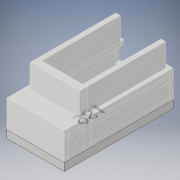
# Autodesk Inventor part: canBusHousing
Saved by Autodesk Inventor 2018.2 (Build 222227000, 227)
## iProperties
Created: 2017-12-01
Part Number: canBusHousing
Material: Generic
Document SubType Name: Modeling
Designer: steele
Density: 1 g/cm^3
Appearance: Default
Author: steele
Autodesk Inventor part; units mm, degrees
ref_plane "YZ Plane" through (0, 0, 0) normal (1, 0, 0) x (0, 1, 0)
ref_plane "XZ Plane" through (0, 0, 0) normal (0, 1, 0) x (-1, 0, 0)
ref_plane "XY Plane" through (0, 0, 0) normal (0, 0, 1) x (1, 0, 0)
sketch "Sketch1" plane through (6.5, -2.85, -13.25) normal (0, -1, 0) x (1, 0, 0)
  line L0 (-6.5, 13.25) -> (-6.5, -0.9821) construction
  line L1 (-6.5, 13.25) -> (1.0035, 13.25) construction
  line L2 (-14.0035, 27.4821) -> (-14.0035, -0.9821)
  line L3 (-14.0035, -0.9821) -> (1.0035, -0.9821)
  line L4 (1.0035, -0.9821) -> (1.0035, 27.4821)
  line L5 (1.0035, 27.4821) -> (-14.0035, 27.4821)
  line L6 (-14.0035, 27.4821) -> (1.0035, -0.9821) construction
  line L7 (-14.0035, -0.9821) -> (1.0035, 27.4821) construction
  constraints: 16 end point, 3 parallel, 2 midpoint, 1 horizontal, 1 perpendicular, 1 vertical
extrude "Extrusion1" add sketch "Sketch1" along normal blind 2
sketch "Sketch2" plane through (6.5, -4.85, -13.25) normal (0, -1, 0) x (1, 0, 0)
  line L0 (1.0035, 27.4821) -> (-14.0035, 27.4821) construction
  line L1 (-8.0035, 27.4821) -> (-8.0035, -0.9797) construction
  line L2 (-14.0035, 27.4821) -> (-14.0035, -0.9821) projected
  spline S0 degree 2 poles (-5.946, 16.5437) (-5.7113, 16.5437) (-5.3211, 16.3906) (-5.1803, 16.2572) knots 0 0 0 1 2 2 2
  spline S1 degree 2 poles (-5.1803, 16.2572) (-5.0444, 16.1312) (-4.8938, 15.7632) (-4.8938, 15.5755) knots 0 0 0 1 2 2 2
  spline S2 degree 2 poles (-4.8938, 15.5755) (-4.8938, 15.3655) (-5.0346, 15.0247) (-5.1679, 14.8987) knots 0 0 0 1 2 2 2
  spline S3 degree 2 poles (-5.1679, 14.8987) (-5.3359, 14.7406) (-5.8793, 14.5677) (-6.2967, 14.5677) knots 0 0 0 1 2 2 2
  spline S4 degree 2 poles (-6.2967, 14.5677) (-6.6747, 14.5677) (-7.3514, 14.7381) (-7.5762, 14.9036) knots 0 0 0 1 2 2 2
  spline S5 degree 2 poles (-7.5762, 14.9036) (-7.8133, 15.079) (-8.0628, 15.573) (-8.0628, 15.9336) knots 0 0 0 1 2 2 2
  spline S6 degree 2 poles (-8.0628, 15.9336) (-8.0628, 16.0151) (-8.0455, 16.2004) (-8.0208, 16.2794) knots 0 0 0 1 2 2 2
  line L3 (-8.0208, 16.2794) -> (-7.6281, 16.2794)
  line L4 (-7.6281, 16.2794) -> (-7.6281, 16.2597)
  spline S7 degree 2 poles (-7.6281, 16.2597) (-7.6577, 16.2078) (-7.7096, 15.9904) (-7.7096, 15.8793) knots 0 0 0 1 2 2 2
  spline S8 degree 2 poles (-7.7096, 15.8793) (-7.7096, 15.4791) (-7.181, 15.0222) (-6.6919, 14.9901) knots 0 0 0 1 2 2 2
  spline S9 degree 2 poles (-6.6919, 14.9901) (-6.8031, 15.1531) (-6.9044, 15.4495) (-6.9044, 15.6249) knots 0 0 0 1 2 2 2
  spline S10 degree 2 poles (-6.9044, 15.6249) (-6.9044, 15.7928) (-6.8303, 16.072) (-6.7241, 16.2127) knots 0 0 0 1 2 2 2
  spline S11 degree 2 poles (-6.7241, 16.2127) (-6.5981, 16.3758) (-6.2152, 16.5437) (-5.946, 16.5437) knots 0 0 0 1 2 2 2
  spline S12 degree 2 poles (-6.2053, 14.9802) (-5.8966, 14.9802) (-5.5063, 15.0938) (-5.4001, 15.1951) knots 0 0 0 1 2 2 2
  spline S13 degree 2 poles (-5.4001, 15.1951) (-5.3013, 15.284) (-5.2272, 15.4693) (-5.2272, 15.5779) knots 0 0 0 1 2 2 2
  spline S14 degree 2 poles (-5.2272, 15.5779) (-5.2272, 15.8299) (-5.5878, 16.1288) (-5.9287, 16.1288) knots 0 0 0 1 2 2 2
  spline S15 degree 2 poles (-5.9287, 16.1288) (-6.1214, 16.1288) (-6.3708, 16.03) (-6.4598, 15.9213) knots 0 0 0 1 2 2 2
  spline S16 degree 2 poles (-6.4598, 15.9213) (-6.524, 15.8422) (-6.566, 15.6471) (-6.566, 15.5335) knots 0 0 0 1 2 2 2
  spline S17 degree 2 poles (-6.566, 15.5335) (-6.566, 15.4026) (-6.4746, 15.1012) (-6.398, 14.9876) knots 0 0 0 1 2 2 2
  spline S18 degree 2 poles (-6.398, 14.9876) (-6.3684, 14.9851) (-6.2671, 14.9802) (-6.2053, 14.9802) knots 0 0 0 1 2 2 2
  spline S19 degree 2 poles (-8.0727, 13.2512) (-8.0727, 13.4784) (-7.9368, 13.8514) (-7.8109, 13.9823) knots 0 0 0 1 2 2 2
  spline S20 degree 2 poles (-7.8109, 13.9823) (-7.6874, 14.1108) (-7.3514, 14.2441) (-7.1612, 14.2441) knots 0 0 0 1 2 2 2
  spline S21 degree 2 poles (-7.1612, 14.2441) (-6.9142, 14.2441) (-6.4993, 13.9798) (-6.3758, 13.7279) knots 0 0 0 1 2 2 2
  line L5 (-6.3758, 13.7279) -> (-6.3634, 13.7279)
  spline S22 degree 2 poles (-6.3634, 13.7279) (-6.2325, 13.9527) (-5.9213, 14.17) (-5.6891, 14.17) knots 0 0 0 1 2 2 2
  spline S23 degree 2 poles (-5.6891, 14.17) (-5.3458, 14.17) (-4.8864, 13.6513) (-4.8864, 13.2512) knots 0 0 0 1 2 2 2
  spline S24 degree 2 poles (-4.8864, 13.2512) (-4.8864, 12.8362) (-5.3211, 12.3348) (-5.6619, 12.3348) knots 0 0 0 1 2 2 2
  spline S25 degree 2 poles (-5.6619, 12.3348) (-5.867, 12.3348) (-6.2671, 12.5744) (-6.3807, 12.7992) knots 0 0 0 1 2 2 2
  line L6 (-6.3807, 12.7992) -> (-6.3931, 12.7992)
  spline S26 degree 2 poles (-6.3931, 12.7992) (-6.5166, 12.5324) (-6.8723, 12.2582) (-7.1538, 12.2582) knots 0 0 0 1 2 2 2
  spline S27 degree 2 poles (-7.1538, 12.2582) (-7.5441, 12.2582) (-8.0727, 12.8264) (-8.0727, 13.2512) knots 0 0 0 1 2 2 2
  spline S28 degree 2 poles (-7.1934, 12.6781) (-7.0056, 12.6781) (-6.7833, 12.8264) (-6.6697, 13.0363) knots 0 0 0 1 2 2 2
  spline S29 degree 2 poles (-6.6697, 13.0363) (-6.6302, 13.1055) (-6.5388, 13.3376) (-6.4795, 13.4834) knots 0 0 0 1 2 2 2
  spline S30 degree 2 poles (-6.4795, 13.4834) (-6.5907, 13.6513) (-6.9217, 13.8316) (-7.1316, 13.8316) knots 0 0 0 1 2 2 2
  spline S31 degree 2 poles (-7.1316, 13.8316) (-7.4082, 13.8316) (-7.7689, 13.4982) (-7.7689, 13.2463) knots 0 0 0 1 2 2 2
  spline S32 degree 2 poles (-7.7689, 13.2463) (-7.7689, 12.9894) (-7.4601, 12.6781) (-7.1934, 12.6781) knots 0 0 0 1 2 2 2
  spline S33 degree 2 poles (-5.6669, 12.735) (-5.4619, 12.735) (-5.1877, 13.0091) (-5.1877, 13.2537) knots 0 0 0 1 2 2 2
  spline S34 degree 2 poles (-5.1877, 13.2537) (-5.1877, 13.476) (-5.4322, 13.76) (-5.6422, 13.76) knots 0 0 0 1 2 2 2
  spline S35 degree 2 poles (-5.6422, 13.76) (-5.7929, 13.76) (-6.0028, 13.6143) (-6.0868, 13.4686) knots 0 0 0 1 2 2 2
  spline S36 degree 2 poles (-6.0868, 13.4686) (-6.1214, 13.4068) (-6.2424, 13.145) (-6.277, 13.0388) knots 0 0 0 1 2 2 2
  spline S37 degree 2 poles (-6.277, 13.0388) (-6.1411, 12.8609) (-5.8521, 12.735) (-5.6669, 12.735) knots 0 0 0 1 2 2 2
  line L7 (-8.0035, 10.1587) -> (-8.0035, 11.6457)
  line L8 (-8.0035, 11.6457) -> (-7.6923, 11.6457)
  line L9 (-7.6923, 11.6457) -> (-7.6923, 11.0924)
  line L10 (-7.6923, 11.0924) -> (-5.6496, 11.0924)
  line L11 (-5.6496, 11.0924) -> (-5.6496, 11.6457)
  line L12 (-5.6496, 11.6457) -> (-5.3705, 11.6457)
  spline S38 degree 2 poles (-5.3705, 11.6457) (-5.3705, 11.332) (-5.1926, 11.0356) (-4.9456, 11.0158) knots 0 0 0 1 2 2 2
  line L13 (-4.9456, 11.0158) -> (-4.9456, 10.6997)
  line L14 (-4.9456, 10.6997) -> (-7.6923, 10.6997)
  line L15 (-7.6923, 10.6997) -> (-7.6923, 10.1587)
  line L16 (-7.6923, 10.1587) -> (-8.0035, 10.1587)
  point P0 (-6.5, 13.25)
  dimension "d2" = 6
  constraints: 2 end point, 2 vertical, 1 point on line
  measures "d2" distance between parallel lines of L2 L1
emboss "Emboss1" sketch "Sketch2" operation cut depth 2 direction (0, 1, 0)
body "Solid1"
